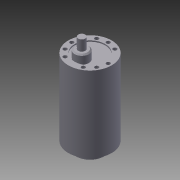
# Autodesk Inventor part: motor
Saved by Autodesk Inventor 2012 (Build 160160000, 160)
## iProperties
Created: 2012-02-28
Part Number: motor
Material: Default
Document SubType Name: Modeling
Designer: Grailas
Density: 1 g/cm^3
Author: Grailas
Autodesk Inventor part; units mm, degrees
ref_plane "YZ Plane" through (0, 0, 0) normal (1, 0, 0) x (0, 1, 0)
ref_plane "XZ Plane" through (0, 0, 0) normal (0, 1, 0) x (-1, 0, 0)
ref_plane "XY Plane" through (0, 0, 0) normal (0, 0, 1) x (1, 0, 0)
sketch "Sketch1" plane through (0, 0, 0) normal (0, 0, 1) x (1, 0, 0)
  circle A0 centre (0, 0) radius 18.4
  circle A1 centre (0, 0) radius 13
  circle A2 centre (0, -7) radius 6
  circle A3 centre (0, -7) radius 3
  circle A4 centre (0, 0) radius 15.5
  circle A5 centre (0, 15.5) radius 1.6
  circle A6 centre (7.75, 13.4234) radius 1.6
  circle A7 centre (-7.75, 13.4234) radius 1.6
  circle A8 centre (-15.5, 0) radius 1.6
  circle A9 centre (-13.4234, -7.75) radius 1.6
  circle A10 centre (-7.75, -13.4234) radius 1.6
  circle A11 centre (15.5, 0) radius 1.6
  circle A12 centre (13.4234, -7.75) radius 1.6
  circle A13 centre (7.75, -13.4234) radius 1.6
  dimension "d0" = 36.8
  dimension "d1" = 6
  dimension "d3" = 12
  dimension "d16" = 3.2
  dimension "d17" = 15.5
  dimension "d19" = 8.0234
  dimension "d20" = 8.0234
  dimension "d21" = 8.0234
  dimension "d22" = 8.0234
  dimension "d25" = 31
  dimension "d26" = 31
  dimension "d27" = 31
  dimension "d28" = 15.5
  dimension "d29" = 15.5
  dimension "d30" = 8.0234
  dimension "d31" = 8.0234
  dimension "d32" = 7
  constraints: 13 centre point, 8 equal radius, 4 coincident, 1 horizontal alignment, 1 tangent, 11 other
  measures "d0" diameter of A0
  measures "d1" diameter of A3
  measures "d3" diameter of A2
  measures "d16" diameter of A5
  measures "d17" distance of A7.centre A8.centre
  measures "d19" distance of A5.centre A7.centre
  measures "d20" distance of A5.centre A6.centre
  measures "d21" distance of A9.centre A8.centre
  measures "d22" distance of A10.centre A9.centre
  measures "d25" distance of A6.centre A10.centre
  measures "d26" distance of A11.centre A8.centre
  measures "d27" distance of A7.centre A13.centre
  measures "d28" distance of A13.centre A10.centre
  measures "d29" distance of A6.centre A11.centre
  measures "d30" distance of A12.centre A11.centre
  measures "d31" distance of A13.centre A12.centre
  measures "d32" distance of point (0, 0) A3.centre
extrude "Extrusion1" add sketch "Sketch1" against normal blind 64.516 contours A0 | A2 | A1 | A3 | A4 A11 | A4 A11 | A11 A4 A12 A13 A10 A9 A8 A7 A5 A6 | A6 A4 | A4 A6 | A12 A4 | A4 A12 | A5 A4 | A4 A5 | A13 A4 | A4 A13 | A7 A4 | A4 A7 | A10 A4 | A4 A10 | A8 A4 | A4 A8 | A9 A4 | A4 A9
extrude "Extrusion2" add sketch "Sketch1" along normal blind 6.5 contours A2
extrude "Extrusion3" add sketch "Sketch1" along normal blind 15.5 contours A3
sketch "Sketch2" plane through (0, 0, -64.516) normal (0, 0, -1) x (-1, 0, 0)
  circle A0 centre (0, 0) radius 18.4 projected
  circle A1 centre (0, 0) radius 12.05
  dimension "d10" = 24.1
  constraints: 1 centre point, 1 coincident
  measures "d10" diameter of A1
extrude "Extrusion4" add sketch "Sketch2" along normal blind 5.6 contours A1
chamfer "Chamfer1" distance 1 angle 45 1 edges at (-6, -7, 6.5)
extrude "Extrusion5" cut sketch "Sketch1" against normal blind 1 contours A1
extrude "Extrusion6" cut sketch "Sketch1" against normal blind 10 contours A4 A11 | A4 A11 | A6 A4 | A4 A6 | A12 A4 | A4 A12 | A5 A4 | A4 A5 | A13 A4 | A4 A13 | A7 A4 | A4 A7 | A10 A4 | A4 A10 | A8 A4 | A4 A8 | A9 A4 | A4 A9
equation "\"d19\" = d20"
equation "\"d21\" = d19"
equation "\"d22\" = d21"
equation "\"d26\" = d25"
equation "\"d27\" = d25"
equation "\"d28\" = d17"
equation "\"d30\" = d19"
body "Solid1"
